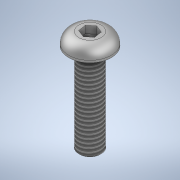
# Autodesk Inventor part: Tornillo Allen cabeza botón M4x16mm
Saved by Autodesk Inventor 2020 (Build 240168000, 168)
## iProperties
Created: 2020-05-08
Part Number: Tornillo Allen cabeza botón M4x16mm
Material: Generic
Document SubType Name: Modeling
Designer: Dante
Density: 1 g/cm^3
Appearance: Rubber - Black - Version 1.1
Mass: 0.335505 g
Surface Area: 3.39406 cm^2
Volume: 0.335505 cm^3
Author: Dante
Autodesk Inventor part; units mm, degrees
ref_plane "YZ Plane" through (0, 0, 0) normal (1, 0, 0) x (0, 1, 0)
ref_plane "XZ Plane" through (0, 0, 0) normal (0, 1, 0) x (-1, 0, 0)
ref_plane "XY Plane" through (0, 0, 0) normal (0, 0, 1) x (1, 0, 0)
sketch "Sketch1" plane through (0, 0, 0) normal (0, 0, 1) x (1, 0, 0)
  line L0 (-9.677, -30.5907) -> (-13.477, -30.5907)
  line L1 (-9.677, -30.5907) -> (-9.677, -46.5907)
  line L2 (-9.677, -46.5907) -> (-11.677, -46.5907)
  line L3 (-11.677, -46.5907) -> (-11.677, -30.5907)
  line L4 (-9.677, -30.5907) -> (-9.677, -26.5988)
  line L5 (-13.477, -30.5907) -> (-13.477, -30.2107)
  line L6 (-13.477, -30.2107) -> (-13.477, -28.3907)
  line L7 (-13.477, -28.3907) -> (-9.677, -28.3907)
  point P0 (0, 0)
  dimension "d0" = 3.8
  dimension "d2" = 16
  dimension "d3" = 2
  dimension "d18" = 0.38
  dimension "d19" = 2.2
  constraints: 16 end point, 3 point on line, 3 vertical, 2 horizontal, 2 perpendicular
  measures "d0" distance of L0.start L0.end
  measures "d2" distance of L0.start L1.end
  measures "d3" distance of L1.end L2.end
  measures "d18" distance of L0.end L5.end
  measures "d19" distance between parallel lines of L0 L7
revolve "Revolution1" add sketch "Sketch1" angle 360 about axis through (-9.677, -30.5907, 0) along (0, -1, 0)
chamfer "Chamfer2" distance 0.2 angle 45 1 edges at (-7.677, -46.5907, 0)
thread "Rosca1" size "M4x0.7" class "6g" standard "ANSI Metric M Profile" full length
fillet "Empalme2" radius 1.82 1 edges at (-5.877, -28.3907, 0)
sketch "Boceto2" plane through (-9.677, -28.3907, 0) normal (0, 1, 0) x (1, 0, 0)
  line L0 (1.1232, 0.9065) -> (1.3467, -0.5194)
  line L1 (1.3467, -0.5194) -> (0.2235, -1.426)
  line L2 (0.2235, -1.426) -> (-1.1232, -0.9065)
  line L3 (-1.1232, -0.9065) -> (-1.3467, 0.5194)
  line L4 (-1.3467, 0.5194) -> (-0.2235, 1.426)
  line L5 (-0.2235, 1.426) -> (1.1232, 0.9065)
  point P0 (9.677, 0)
  point P1 (0, 0)
  dimension "d21" = 2.5
  constraints: 12 end point, 13 other
  measures "d21" distance between parallel lines of L1 L4
extrude "Extrusión1" cut sketch "Boceto2" against normal blind 1.3
body "Solid1"
